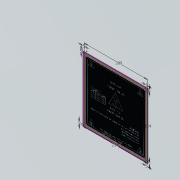
# Autodesk Inventor part: HeatedBed
Saved by Autodesk Inventor 2016 (Build 200138000, 138)
## iProperties
Created: 2016-08-03
Part Number: HeatedBed
Material: Generic
Document SubType Name: Modeling
Designer: Sam
Density: 1 g/cm^3
Appearance: Default
Author: Sam
Autodesk Inventor part; units mm, degrees
ref_plane "YZ Plane" through (0, 0, 0) normal (1, 0, 0) x (0, 1, 0)
ref_plane "XZ Plane" through (0, 0, 0) normal (0, 1, 0) x (-1, 0, 0)
ref_plane "XY Plane" through (0, 0, 0) normal (0, 0, 1) x (1, 0, 0)
sketch "Sketch1" plane through (0, 0, 0) normal (0, 1, 0) x (-1, 0, 0)
  line L0 (12.8073, -5) -> (-201.1927, -5)
  line L1 (-201.1927, -5) -> (-201.1927, -219)
  line L2 (-201.1927, -219) -> (12.8073, -219)
  line L3 (12.8073, -219) -> (12.8073, -5)
  line L4 (-194.2832, -13.9005) -> (3.3163, -13.9005) construction
  line L5 (3.3163, -13.9005) -> (3.3163, -210.6364) construction
  line L6 (3.3163, -210.6364) -> (-194.2832, -210.6364) construction
  line L7 (-194.2832, -210.6364) -> (-194.2832, -13.9005) construction
  point P0 (0, 0)
  point P1 (7.8073, -10)
  point P2 (7.8073, -214)
  point P3 (-196.1927, -214)
  point P4 (-196.1927, -10)
  dimension "d0" = 214
  dimension "d1" = 214
  dimension "d2" = 209
  dimension "d3" = 5
  dimension "d4" = 5
  dimension "d5" = 5
  dimension "d6" = 5
  dimension "d7" = 5
  dimension "d8" = 5
  dimension "d9" = 5
  constraints: 8 end point, 2 parallel, 1 horizontal, 1 perpendicular, 2 other
  measures "d0" distance of L2.end L1.end
  measures "d1" distance of L1.end L0.end
  measures "d2" distance from line of L1 point (7.807, -10)
  measures "d3" distance from line of L3 point (7.807, -214)
  measures "d4" distance from line of L2 point (7.807, -214)
  measures "d5" distance from line of L0 point (7.807, -10)
  measures "d6" distance from line of L1 point (-196.193, -10)
  measures "d7" distance from line of L0 point (-196.193, -10)
  measures "d8" distance from line of L2 point (-196.193, -214)
  measures "d9" distance from line of L1 point (-196.193, -214)
extrude "Extrusion1" add sketch "Sketch1" along normal blind 3
hole "Hole1" at (-7.8073, 0, -10) at (-7.8073, 0, -214) at (196.1927, 0, -214) at (196.1927, 0, -10) direction (0, 1, 0) diameter 3.2 end through all
body "Solid1"
